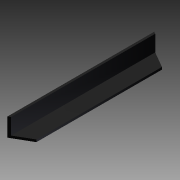
# Autodesk Inventor part: angle template al-6061 1x1x0.125
Saved by Autodesk Inventor 2012 (Build 160160000, 160)
## iProperties
Created: 2011-11-26
Part Number: angle template al-6061 1x1x0.125
Material: Aluminum-6061
Document SubType Name: Modeling
Designer: Antonella
Mass: 249.8 g
Surface Area: 622.378 cm^2
Volume: 92.1772 cm^3
Density: 2.71 g/cm^3
Author: Antonella
Autodesk Inventor part; units mm, degrees
ref_plane "YZ Plane" through (0, 0, 0) normal (1, 0, 0) x (0, 1, 0)
ref_plane "XZ Plane" through (0, 0, 0) normal (0, 1, 0) x (-1, 0, 0)
ref_plane "XY Plane" through (0, 0, 0) normal (0, 0, 1) x (1, 0, 0)
sketch "Sketch1" plane through (0, 0, 0) normal (0, 0, 1) x (1, 0, 0)
  line L0 (-17.78, 0) -> (17.78, 0) projected
  line L1 (0, -17.78) -> (0, 17.78) projected
  line L2 (-12.7, 12.7) -> (-12.7, -12.7)
  line L3 (-12.7, -12.7) -> (12.7, -12.7)
  line L4 (12.7, -9.525) -> (-9.525, -9.525)
  line L5 (-9.525, -9.525) -> (-9.525, 12.7)
  line L6 (-12.7, 12.7) -> (-9.525, 12.7)
  line L7 (12.7, -12.7) -> (12.7, -9.525)
  point P0 (0, 0)
  point P1 (-12.7, 0)
  point P2 (0, -12.7)
  dimension "d0" = 25.4
  dimension "d1" = 3.175
  constraints: 12 end point, 5 perpendicular, 2 midpoint, 1 horizontal alignment, 1 parallel, 1 vertical alignment, 1 other
  measures "d0" distance of L2.start L2.end
  measures "d1" distance between parallel lines of L4 L3
extrude "Extrusion1" add sketch "Sketch1" along normal mid plane 203.2 contours L2 L6 L5 L0 | L0 L5 L4 L1 L3 L2 | L1 L4 L7 L3
sketch "Sketch2" plane through (-9.525, -9.525, 101.6) normal (0, 1, 0) x (1, 0, 0)
  line L0 (22.225, 203.2) -> (22.225, 0) projected
  line L1 (22.225, 203.2) -> (0, 203.2) projected
  line L2 (-3.175, 0) -> (-3.175, 203.2) projected
  line L3 (-3.175, 203.2) -> (22.225, 188.5353)
  line L4 (22.225, 101.6) -> (-3.175, 101.6) construction
  line L5 (0, 203.2) -> (-3.175, 203.2) projected
  line L6 (-3.175, 0) -> (0, 0) projected
  line L7 (22.225, 188.5353) -> (22.225, 203.2)
  line L8 (22.225, 203.2) -> (-3.175, 203.2)
  line L9 (-3.175, 0) -> (22.225, 14.6647)
  line L10 (22.225, 14.6647) -> (22.225, 0)
  line L11 (22.225, 0) -> (-3.175, 0)
  point P0 (9.525, 101.6)
  dimension "d4" = 30
  dimension "d5" = 30
  constraints: 14 end point, 4 perpendicular, 2 midpoint, 2 point on line
  measures "d4" angle of L1 L3
  measures "d5" angle of L9 L11
extrude "Extrusion2" cut sketch "Sketch2" along normal through all both and the other way through all contours L0 L3 L5 L1 | L0 L11 L6 L9
body "Solid1"
